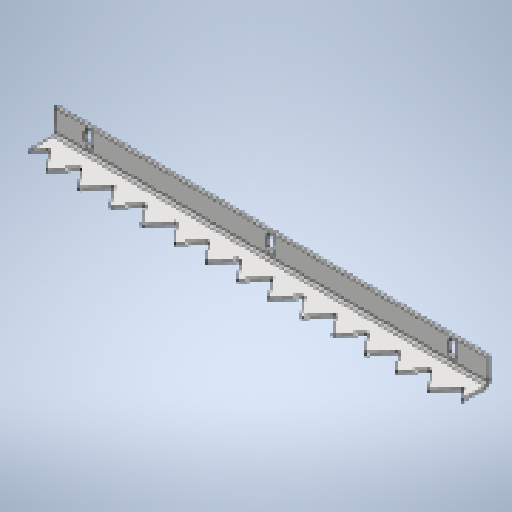
# Autodesk Inventor part: TRM 34 comb 3
Saved by Autodesk Inventor 2025.1 (Build 291241020, 241B)
## iProperties
Created: 2024-08-07
Part Number: TRM 34 comb 3
Material: AISI 304
Document SubType Name: Sheet Metal
Designer: user
Stock Number: ТРМ 018 отсекатель
Density: 8.02768 g/cm^3
Flat Pattern Width: 6.46266 cm
Flat Pattern Length: 47.6 cm
Flat Pattern Area: 307.623 cm^2
Sheet Metal Rule: AISI304 2mm Die16
Sheet Metal Width: 64.627 mm
Sheet Metal Length: 476.000 mm
Sheet Metal Area: 30762.267 mm^2
Appearance: Default
Author: pokla
Autodesk Inventor part; units mm, degrees
ref_plane "YZ Plane" through (0, 0, 0) normal (1, 0, 0) x (0, 1, 0)
ref_plane "XZ Plane" through (0, 0, 0) normal (0, 1, 0) x (-1, 0, 0)
ref_plane "XY Plane" through (0, 0, 0) normal (0, 0, 1) x (1, 0, 0)
sketch "Sketch1" plane through (0, 0, 0) normal (0, 0, 1) x (1, 0, 0)
  line L0 (-238, -20) -> (238, -20)
  line L1 (238, -20) -> (238, 20)
  line L2 (238, 20) -> (-238, 20)
  line L3 (-238, 20) -> (-238, -20)
  line L4 (-238, -20) -> (238, 20) construction
  line L5 (238, -20) -> (-238, 20) construction
  point P0 (0, 0)
  dimension "d0" = 476
  dimension "d1" = 40
  measures "d0" distance of L2.end L1.end
  measures "d1" distance of L1.end L0.end
extrude "Plate1" add sketch "Sketch1" along normal blind 3
sketch "Sketch6" plane through (0, 0, 3) normal (0, 0, 1) x (1, 0, 0)
  line L0 (238, -20) -> (-238, -20) projected
  line L1 (238, 20) -> (238, -20) projected
  line L2 (-238, 20) -> (238, 20) projected
  line L3 (-238, -20) -> (-238, 20) projected
  line L4 (15.8465, 0) -> (18.8465, 0)
  line L5 (18.8465, 0) -> (34.1931, -20)
  line L6 (15.8465, 0) -> (0.5, -20)
  line L7 (238, -20) -> (-238, -20) projected
  point P0 (0, 0)
  point P1 (17.3465, 0)
  point P2 (0, -20)
  point P3 (0, -20)
  dimension "d33" = 20
  dimension "d35" = 3
  dimension "d81" = 0.5
  dimension "d82" = 75
  constraints: 6 end point, 3 midpoint, 2 point on line, 1 equal length, 1 horizontal
  measures "d33" distance between parallel lines of L0 L4
  measures "d35" distance of L4.start L4.end
  measures "d81" distance of point (0, -20) L6.end
  measures "d82" angle of L6 L5
extrude "Cut1" cut sketch "Sketch6" against normal blind 3 contours L0 L6 L4 L5
pattern_linear "Rectangular Pattern1" count 44 spacing 35 along (-1, 0, 0) of "Cut1" first direction both ways yes
sketch "Sketch7" plane through (-238, 17.0018, -0.1047) normal (0, 0.9993908, 0.0348995) x (-1, 0, 0)
  line L0 (-476, 0) -> (0, 0)
  line L1 (0, 0) -> (0, 30)
  line L2 (0, 30) -> (-476, 30)
  line L3 (-476, 30) -> (-476, 0)
  constraints: 6 end point, 1 horizontal, 1 perpendicular, 1 vertical
edge flange "Flange3" height 30 angle 92 thickness 3 bend radius 2.75 thickness toward (0, 0.9993908, 0.0348995) relief round relief width 3 relief depth 1.5 edges at (0, 20, 3) wall of the first edge with corners at (238, 17.0018, -0.1047) (-238, 17.0018, -0.1047) (-238, 15.9548, 29.877) (238, 15.9548, 29.877)
bend "Bend3"
corner "Corner3"
sketch "Sketch8" plane through (-238, 18.953, 29.9817) normal (0, 0.9993908, 0.0348995) x (1, 0, 0)
  line L0 (238, 17) -> (238, 7) construction
  line L1 (233.5, 17) -> (233.5, 7)
  line L2 (242.5, 7) -> (242.5, 17)
  arc A0 (242.5, 17) -> (233.5, 17) centre (238, 17) ccw
  arc A1 (233.5, 7) -> (242.5, 7) centre (238, 7) ccw
  line L3 (476, 0) -> (0, 0) projected
  point P0 (238, 29.302)
  point P1 (238, 12)
  dimension "d51" = 9
  dimension "d53" = 10
  dimension "d79" = 7
  constraints: 8 end point, 4 point on circle, 4 tangent, 2 centre point, 1 midpoint, 1 parallel, 1 vertical, 1 vertical alignment
  measures "d51" diameter of A1
  measures "d53" distance of L0.start L0.end
  measures "d79" distance from line of L0.end L3
extrude "Cut2" cut sketch "Sketch8" against normal blind 3
pattern_linear "Rectangular Pattern2" count 3 spacing 200 along (-1, 0, 0) of "Cut2" first direction both ways yes
equation "\"d36\" = Thickness"
equation "\"d54\" = Thickness"
equation "\"d2\" = Thickness"
equation "\"d41\" = BendReliefWidth"
equation "\"d42\" = BendReliefDepth"
equation "\"d43\" = MinimumRemnant"
equation "\"d44\" = TransitionRadius"
equation "\"d47\" = BendRadius"
equation "\"d48\" = CornerReliefSize"
equation "\"d49\" = GapSize"
equation "\"d50\" = JacobiRadiusSize"
equation "\"BendReliefWidth\" = Thickness"
equation "\"BendReliefDepth\" = 0.5 * Thickness"
equation "\"CornerReliefSize\" = 4 * Thickness"
equation "\"MinimumRemnant\" = 2 * Thickness"
equation "\"TransitionRadius\" = BendRadius"
equation "\"JacobiRadiusSize\" = BendRadius"
equation "\"GapSize\" = Thickness"
equation "\"Thickness\" = 3"
equation "\"BendRadius\" = 2.75"
body "Solid1"
